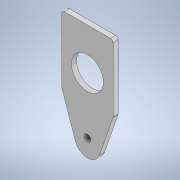
# Autodesk Inventor part: Frame1
Saved by Autodesk Inventor 2020 (Build 240168000, 168)
## iProperties
Created: 2022-06-23
Part Number: Frame1
Material: Generic
Document SubType Name: Modeling
Designer: karimi2
Density: 1 g/cm^3
Appearance: Default
Author: karimi2
Autodesk Inventor part; units mm, degrees
ref_plane "YZ Plane" through (0, 0, 0) normal (1, 0, 0) x (0, 1, 0)
ref_plane "XZ Plane" through (0, 0, 0) normal (0, 1, 0) x (-1, 0, 0)
ref_plane "XY Plane" through (0, 0, 0) normal (0, 0, 1) x (1, 0, 0)
sketch "Sketch1" plane through (0, 0, 0) normal (0, 0, 1) x (1, 0, 0)
  line L0 (0, 0) -> (0, 100) construction
  line L1 (0, 90) -> (-20, 90)
  line L2 (-20, 90) -> (-20, 37.5)
  arc A0 (-9.4595, 6.7568) -> (0, 0) centre (0, 10) ccw
  line L3 (-20, 37.5) -> (-9.4595, 6.7568)
  line L4 (0, 90) -> (20, 90)
  line L5 (20, 90) -> (20, 37.5)
  arc A1 (0, 0) -> (9.4595, 6.7568) centre (0, 10) ccw
  line L6 (20, 37.5) -> (9.4595, 6.7568)
  circle A2 centre (0, 57.5) radius 12.5
  circle A3 centre (0, 13.5) radius 2.6
  dimension "d2" = 20
  dimension "d4" = 52.5
  dimension "d5" = 37.5
  dimension "d6" = 10
  dimension "d7" = 32.5
  dimension "d8" = 25
  dimension "d9" = 13.5
  dimension "d10" = 5.2
  constraints: 14 end point, 4 centre point, 4 point on circle, 4 point on line, 3 symmetric about line, 2 vertical, 1 horizontal, 1 tangent, 1 other
  measures "d2" distance of L1.start L1.end
  measures "d4" distance of L1.end L2.end
  measures "d5" vertical distance of L0.start L2.end
  measures "d6" distance of L0.start A0.centre
  measures "d7" distance of L1.start A2.centre
  measures "d8" diameter of A2
  measures "d9" distance of L0.start A3.centre
  measures "d10" diameter of A3
extrude "Extrusion1" add sketch "Sketch1" along normal mid plane 4
fillet "Fillet1" radius 2 5 edges at (20, 37.5, 0) (20, 90, 0) (-20, 90, 0) (-20, 37.5, 1) (-20, 37.5, -1)
body "Solid1"
